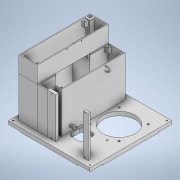
# Autodesk Inventor part: Spód
Saved by Autodesk Inventor 2022 (Build 260153000, 153)
## iProperties
Created: 2022-07-08
Part Number: Spód
Material: Ogólny
Document SubType Name: Modeling
Designer: kosak
Density: 1 g/cm^3
Appearance: Domyślna
Mass: 628.246 g
Surface Area: 3320.76 cm^2
Volume: 628.246 cm^3
Author: kosak
## iProperties of the stored document Base_Drukowanie 3D.ipt
Created: 2022-07-14
Part Number: Base_Drukowanie 3D
Material: Ogólny
Document SubType Name: Modeling
Designer: kosak
Density: 1 g/cm^3
Appearance: Domyślna
Author: kosak
Autodesk Inventor part; units mm, degrees
(part 1 of 2)
ref_plane "YZ Plane" through (0, 0, 0) normal (1, 0, 0) x (0, 1, 0)
ref_plane "XZ Plane" through (0, 0, 0) normal (0, 1, 0) x (-1, 0, 0)
ref_plane "XY Plane" through (0, 0, 0) normal (0, 0, 1) x (1, 0, 0)
sketch "Podstawa" plane through (0, 0, 0) normal (0, 1, 0) x (-1, 0, 0)
  line L0 (0, 0) -> (200, 0)
  line L1 (200, 0) -> (200, -200)
  line L2 (200, -200) -> (0, -200)
  line L3 (0, -200) -> (0, 0)
  dimension "d0" = 200
  dimension "d1" = 200
  constraints: 8 end point, 2 parallel, 1 horizontal, 1 perpendicular
  measures "d0" distance of L1.end L2.end
  measures "d1" distance of L0.end L1.end
extrude "Wyciągnięcie proste1" add sketch "Podstawa" against normal blind 10
ref_plane "Płaszczyzna konstrukcyjna3" through (0, 0, 0) normal (0, 1, 0) x (1, 0, 0)
sketch "Obrys" plane through (0, 0, 0) normal (0, 1, 0) x (1, 0, 0)
  line L0 (-200, 200) -> (0, 200) projected
  line L1 (0, 200) -> (0, 0) projected
  line L2 (-200, 200) -> (0, 200)
  line L3 (0, 200) -> (0, 0)
  line L4 (0, 0) -> (-200, 0)
  line L5 (-200, 0) -> (-200, 200)
  line L6 (-190, 190) -> (-10, 190)
  line L7 (-10, 190) -> (-10, 10)
  line L8 (-10, 10) -> (-190, 10)
  line L9 (-190, 10) -> (-190, 190)
  line L10 (-200, 0) -> (-200, 200) projected
  line L11 (-190, 190) -> (-100, 190)
  line L12 (-100, 190) -> (-96.5, 190)
  line L13 (-100, 190) -> (-103.5, 190)
  line L14 (-96.5, 190) -> (-94.2905, 190)
  line L15 (-103.5, 190) -> (-106.0324, 190)
  line L16 (-96.5, 190) -> (-103.5, 190)
  line L17 (-103.5, 190) -> (-103.5, 10)
  line L18 (-103.5, 10) -> (-96.5, 10)
  line L19 (-96.5, 10) -> (-96.5, 190)
  dimension "d5" = 10
  constraints: 34 end point, 6 parallel, 5 point on line, 3 perpendicular, 2 horizontal, 1 midpoint, 3 other
  measures "d5" distance between parallel lines of L5 L9
extrude "Wyciągnięcie proste2" [suppressed]
sketch "Podstawa - kanał powietrzny" plane through (0, 0, 0) normal (0, 1, 0) x (1, 0, 0)
  line L0 (-187, 13) -> (-187, 187)
  line L1 (-187, 187) -> (-100, 187)
  line L2 (-95.5, 13) -> (-187, 13)
  line L3 (-187, 187) -> (-142.5, 187)
  line L4 (-142.5, 187) -> (-142.5, 142.5)
  line L5 (-142.5, 142.5) -> (-187, 142.5)
  line L6 (-187, 142.5) -> (-187, 187)
  line L7 (-187, 13) -> (-142.5, 13)
  line L8 (-142.5, 13) -> (-142.5, 57.5)
  line L9 (-142.5, 57.5) -> (-187, 57.5)
  line L10 (-187, 57.5) -> (-187, 13)
  line L11 (-185, 185) -> (-144.5, 185)
  line L12 (-144.5, 185) -> (-144.5, 144.5)
  line L13 (-144.5, 144.5) -> (-185, 144.5)
  line L14 (-185, 144.5) -> (-185, 185)
  line L15 (-185, 55.5) -> (-144.5, 55.5)
  line L16 (-144.5, 55.5) -> (-144.5, 15)
  line L17 (-144.5, 15) -> (-185, 15)
  line L18 (-185, 15) -> (-185, 55.5)
  line L19 (-190, 190) -> (-190, 10) projected
  line L20 (-190, -20.8628) -> (-103.5, -20.8628)
  line L21 (-10, 10) -> (-190, 10) projected
  line L22 (-103.5, 10) -> (-103.5, 190)
  line L23 (-10, 190) -> (-190, 190) projected
  line L24 (-97.8, 10) -> (-189, 10)
  line L25 (-187, 13) -> (-10, 13)
  line L26 (-200, 0) -> (-200, 200) projected
  line L27 (-200, 200) -> (0, 200) projected
  line L28 (0, 200) -> (0, 0) projected
  line L29 (0, 0) -> (-200, 0) projected
  point P0 (-142.5, 187)
  point P1 (-142.5, 13)
  point P2 (-142.5, 13)
  dimension "d23" = 44.5
  dimension "d24" = 44.5
  dimension "d25" = 44.5
  dimension "d27" = 2
  dimension "d28" = 2
  dimension "d34" = 86.5
  dimension "d132" = 44.5
  constraints: 46 end point, 10 parallel, 5 perpendicular, 3 horizontal, 3 point on line, 1 collinear, 6 other
  measures "d23" distance of L4.end L5.end
  measures "d24" distance of L3.end L4.end
  measures "d25" distance of L9.end L8.end
  measures "d27" distance between parallel lines of L6 L14
  measures "d28" distance between parallel lines of L9 L15
  measures "d34" distance of L20.start L20.end
  measures "d132" distance between parallel lines of L9 L2
extrude "Wyciągnięcie proste5" add sketch "Podstawa - kanał powietrzny" along normal blind 100 and the other way blind 10 contours L0 L9 L8 L2 | L0 L1 L4 L5
sketch "Szkic7" plane through (0, 0, 0) normal (0, 1, 0) x (1, 0, 0)
  line L0 (-185, 144.5) -> (-144.5, 144.5) projected
  line L1 (-144.5, 144.5) -> (-144.5, 185) projected
  line L2 (-144.5, 185) -> (-185, 185) projected
  line L3 (-185, 185) -> (-185, 144.5) projected
  line L4 (-187, 142.5) -> (-187, 187) projected
  line L5 (-187, 187) -> (-142.5, 187) projected
  line L6 (-142.5, 187) -> (-142.5, 142.5) projected
  line L7 (-142.5, 142.5) -> (-187, 142.5) projected
  line L8 (-185, 15) -> (-144.5, 15) projected
  line L9 (-144.5, 15) -> (-144.5, 55.5) projected
  line L10 (-144.5, 55.5) -> (-185, 55.5) projected
  line L11 (-185, 55.5) -> (-185, 15) projected
  line L12 (-142.5, 57.5) -> (-142.5, 13) projected
  line L13 (-187, 13) -> (-187, 57.5) projected
  line L14 (-187, 57.5) -> (-142.5, 57.5) projected
  line L15 (-187, 13) -> (-187, 187)
  line L16 (-187, 187) -> (-100.8544, 187)
  line L17 (-100.8544, 13) -> (-187, 13)
  line L18 (-184.5, 142.5) -> (-184.5, 57.5)
  line L19 (-100.8544, 187) -> (-100.8544, 13)
  line L20 (-103.5, 10) -> (-96.5, 10) projected
  line L21 (-103.5, 13) -> (-100.8544, 13)
  line L22 (-103.5, 187) -> (-100.8544, 187)
  line L23 (-142.5, 142.5) -> (-187, 142.5) projected
  line L24 (-184.5, 142.5) -> (-142.5, 142.5)
  line L25 (-142.5, 142.5) -> (-142.5, 187)
  line L26 (-100.8544, 187) -> (-100.8544, 13)
  line L27 (-187, 57.5) -> (-142.5, 57.5) projected
  line L28 (-142.5, 57.5) -> (-184.5, 57.5)
  line L29 (-142.5, 13) -> (-187, 13) projected
  line L30 (-187, 13) -> (-142.5, 13) projected
  line L31 (-200, 0) -> (-200, 200) projected
  line L32 (-200, 200) -> (0, 200) projected
  line L33 (0, 200) -> (0, 0) projected
  line L34 (0, 0) -> (-200, 0) projected
  point P0 (-142.5, 13)
  point P1 (-142.5, 187)
  point P2 (-187, 57.5)
  constraints: 22 end point, 4 collinear, 4 point on line, 1 perpendicular
sketch "Otwory spód - kanał pow." plane through (0, -10, 0) normal (0, -1, 0) x (1, 0, 0)
  line L0 (-185, -144.5) -> (-144.5, -144.5) projected
  line L1 (-185, -185) -> (-185, -144.5) projected
  line L2 (-144.5, -185) -> (-185, -185) projected
  line L3 (-144.5, -144.5) -> (-144.5, -185) projected
  line L4 (-185, -55.5) -> (-185, -15) projected
  line L5 (-144.5, -55.5) -> (-185, -55.5) projected
  line L6 (-185, -15) -> (-144.5, -15) projected
  line L7 (-144.5, -15) -> (-144.5, -55.5) projected
  line L8 (-144.5, -185) -> (-185, -185) projected
  line L9 (-185, -185) -> (-144.5, -185)
  line L10 (-144.5, -185) -> (-144.5, -144.5)
  line L11 (-144.5, -144.5) -> (-185, -144.5)
  line L12 (-185, -144.5) -> (-185, -185)
  line L13 (-185, -55.5) -> (-144.5, -55.5) projected
  line L14 (-185, -55.5) -> (-144.5, -55.5)
  line L15 (-144.5, -55.5) -> (-144.5, -15)
  line L16 (-144.5, -15) -> (-185, -15)
  line L17 (-185, -15) -> (-185, -55.5)
  constraints: 16 end point, 4 parallel, 2 horizontal, 2 perpendicular
extrude "Otwory - spód" cut sketch "Otwory spód - kanał pow." against normal blind 10
ref_plane "Płaszczyzna konstrukcyjna4" through (-189, 0, -188) normal (0, 0, 1) x (1, 0, 0)
extrude "Wyciągnięcie proste18" add sketch "Szkic7" along normal blind 100 separate body contours L7 L18 L14 L15 | L7 L6 L16 L19 L17 L12 L14 L18 | L14 L12 L17 L13 | L11 L10 L9 L8
sketch "Szkic34" plane through (-142.5, 0, -187) normal (0, 0, -1) x (-1, 0, 0)
  line L0 (44.5, 0) -> (44.5, 100) projected
  line L1 (-142.5, 0.5) -> (57.5, 0.5) projected
  line L2 (44.5, 0.5) -> (32.5, 0.5)
  line L3 (32.5, 0.5) -> (32.5, 12.5)
  line L4 (32.5, 12.5) -> (44.5, 12.5)
  line L5 (44.5, 12.5) -> (44.5, 0.5)
  point P0 (-142.5, 0)
  point P1 (42.5, 201)
  point P2 (44.3955, 10.5)
  point P3 (32.5, 0.5)
  point P4 (44.5, 140)
  point P5 (44.5, 12.5)
  point P6 (44.5, 1)
  point P7 (44.5, 12.5)
  dimension "d113" = 12
  dimension "d114" = 12
  constraints: 8 end point, 2 parallel, 1 horizontal, 1 perpendicular, 1 point on line, 2 other
  measures "d113" distance of L3.end L4.end
  measures "d114" distance of L2.end L3.end
extrude "Kanał wodny - mały spód" add sketch "Szkic34" against normal blind 42.5 bodies 1
sketch "Szkic33" plane through (-142.5, 0, -187) normal (0, 0, -1) x (-1, 0, 0)
  line L0 (-142.5, 0.5) -> (57.5, 0.5) projected
  line L1 (44.5, 0) -> (44.5, 100) projected
  line L2 (47.5, 0.5) -> (-132.5, 0.5) projected
  line L3 (-132.5, 0.5) -> (47.5, 0.5) projected
  line L4 (44.5, 0.5) -> (32.5, 0.5)
  line L5 (32.5, 0.5) -> (32.5, 12.5)
  line L6 (32.5, 12.5) -> (44.5, 12.5)
  line L7 (44.5, 12.5) -> (44.5, 0.5)
  line L8 (42.5, 10.5) -> (34.5, 10.5)
  line L9 (34.5, 10.5) -> (34.5, 2.5)
  line L10 (34.5, 2.5) -> (42.5, 2.5)
  line L11 (42.5, 2.5) -> (42.5, 10.5)
  point P0 (-142.5, 0)
  point P1 (42.5, 201)
  point P2 (-43, 0.5)
  point P3 (44.5, 140)
  point P4 (44.5, 1)
  dimension "d108" = 12
  dimension "d109" = 12
  dimension "d110" = 2
  constraints: 16 end point, 4 parallel, 2 perpendicular, 1 horizontal, 1 point on line, 5 other
  measures "d108" distance of L5.end L6.end
  measures "d109" distance of L4.end L5.end
  measures "d110" distance between parallel lines of L6 L8
extrude "Kanał wodny - mały, spód" cut sketch "Szkic33" against normal blind 42.5 contours L11 L10 L9 L8 bodies 1
sketch "Szkic39" plane through (0, 100, 0) normal (0, 1, 0) x (1, 0, 0)
  line L0 (-144.5, 55.5) -> (-185, 55.5) projected
  line L1 (-185, 15) -> (-144.5, 15) projected
  line L2 (-185, 55.5) -> (-144.5, 55.5)
  line L3 (-144.5, 55.5) -> (-144.5, 15)
  line L4 (-144.5, 15) -> (-185, 15)
  line L5 (-185, 15) -> (-185, 55.5)
  point P0 (0, 0)
  point P1 (-170, 15)
  point P2 (-170, 15)
  constraints: 8 end point, 2 parallel, 1 horizontal, 1 perpendicular
extrude "Wyciągnięcie proste30" cut sketch "Szkic39" against normal blind 110 bodies 2
ref_plane "Płaszczyzna konstrukcyjna10" through (-164.75, 100, -15) normal (0, 1, 0) x (1, 0, 0)
sketch "Szkic40" plane through (-164.75, 100, -15) normal (0, 1, 0) x (1, 0, 0)
  line L0 (-22.25, 42.5) -> (-22.25, -2) projected
  line L1 (22.25, 127.5) -> (22.25, 172) projected
  line L2 (-22.25, -2) -> (22.25, -2)
  line L3 (22.25, -2) -> (22.25, 172)
  line L4 (22.25, 172) -> (-22.25, 172)
  line L5 (-22.25, 172) -> (-22.25, -2)
  point P0 (164.75, -15)
  constraints: 8 end point, 2 parallel, 1 horizontal, 1 perpendicular
extrude "Wyciągnięcie proste31" add sketch "Szkic40" along normal blind 40 bodies 2
sketch "Szkic41" plane through (-187, 0, -13) normal (0, 0, 1) x (1, 0, 0)
  line L0 (0, 140) -> (44.5, 140) projected
  line L1 (44.5, 100) -> (44.5, 140) projected
  line L2 (0, 100) -> (44.5, 100) projected
  line L3 (0, 102) -> (42.5, 102)
  line L4 (42.5, 102) -> (42.5, 138)
  line L5 (42.5, 138) -> (0, 138)
  line L6 (0, 138) -> (2, 138)
  line L7 (2, 138) -> (2, 102)
  line L8 (42.5, 102) -> (2, 102)
  line L9 (2, 102) -> (2, 138)
  line L10 (2, 138) -> (42.5, 138)
  line L11 (42.5, 138) -> (42.5, 102)
  point P0 (187, 0)
  dimension "d137" = 2
  dimension "d138" = 2
  constraints: 18 end point, 2 parallel, 2 perpendicular, 2 point on line, 1 horizontal, 2 other
  measures "d137" distance between parallel lines of L2 L3
  measures "d138" distance of L5.end L6.end
extrude "Wyciągnięcie proste32" cut sketch "Szkic41" against normal blind 172 bodies 2
sketch "Szkic42" plane through (-185, 102, -13) normal (0, 1, 0) x (1, 0, 0)
  line L0 (40.5, 2) -> (0, 2) projected
  line L1 (0, 0) -> (0, 172) projected
  line L2 (40.5, 0) -> (40.5, 172) projected
  line L3 (0, 42.5) -> (40.5, 42.5) projected
  line L4 (40.5, 42.5) -> (0, 42.5) projected
  line L5 (40.5, 2) -> (40.5, 42.5) projected
  line L6 (0, 42.5) -> (40.5, 42.5)
  line L7 (40.5, 42.5) -> (40.5, 2)
  line L8 (40.5, 2) -> (0, 2)
  line L9 (0, 2) -> (0, 42.5)
  line L10 (40.5, 131.5) -> (0, 131.5) projected
  line L11 (40.5, 172) -> (0, 172) projected
  line L12 (40.5, 131.5) -> (40.5, 172) projected
  line L13 (0, 172) -> (0, 131.5) projected
  line L14 (40.5, 172) -> (0, 172)
  line L15 (0, 172) -> (0, 131.5)
  line L16 (0, 131.5) -> (40.5, 131.5)
  line L17 (40.5, 131.5) -> (40.5, 172)
  point P0 (185, -13)
  point P1 (0, 157)
  constraints: 16 end point, 4 parallel, 2 horizontal, 2 perpendicular
extrude "Wyciągnięcie proste34" cut sketch "Szkic42" against normal blind 110 contours L0 L1 L3 L2 | L10 L1 L11 L2 bodies 2
sketch "Szkic44" plane through (0, 100, 0) normal (0, 1, 0) x (1, 0, 0)
  line L0 (-144.5, 55.5) -> (-144.5, 15) projected
  line L1 (-142.5, 13) -> (-100.8544, 13) projected
  line L2 (-100.8544, 13) -> (-100.8544, 187) projected
  line L3 (-100.8544, 187) -> (-142.5, 187) projected
  line L4 (-144.5, 185) -> (-144.5, 144.5) projected
  line L5 (-144.5, 144.5) -> (-185, 144.5) projected
  line L6 (-187, 142.5) -> (-187, 13) projected
  line L7 (-185, 55.5) -> (-144.5, 55.5) projected
  line L8 (-142.5, 185) -> (-102.8544, 185)
  line L9 (-102.8544, 185) -> (-102.8544, 15)
  line L10 (-102.8544, 15) -> (-142.5, 15)
  line L11 (-142.5, 15) -> (-142.5, 55.5)
  line L12 (-142.5, 142.5) -> (-142.5, 13) projected
  line L13 (-187, 57.5) -> (-142.5, 57.5) projected
  line L14 (-185, 57.5) -> (-142.5, 57.5)
  line L15 (-142.5, 57.5) -> (-142.5, 56.1633)
  line L16 (-185, 57.5) -> (-185, 142.5)
  line L17 (-142.5, 142.5) -> (-187, 142.5) projected
  line L18 (-185, 142.5) -> (-142.5, 142.5)
  line L19 (-142.5, 142.5) -> (-142.5, 185)
  line L20 (-142.5, 187) -> (-142.5, 142.5) projected
  point P0 (0, 0)
  dimension "d149" = 2
  constraints: 18 end point, 4 point on line, 2 collinear, 1 parallel, 1 perpendicular, 2 other
  measures "d149" distance between parallel lines of L2 L9
extrude "Wyciągnięcie proste36" cut sketch "Szkic44" against normal blind 100 contours L11 L12 L19 L8 L9 L10 | L13 L16 L17 L12 bodies 2
ref_plane "Płaszczyzna konstrukcyjna18" through (-164.75, 293.9, -15) normal (0, 1, 0) x (1, 0, 0)
sketch "Szkic49" plane through (-164.75, 293.9, -15) normal (0, 1, 0) x (1, 0, 0)
  line L0 (-22.25, 160) -> (-10.25, 160) projected
  line L1 (-10.25, 160) -> (-10.25, 172) projected
  line L2 (-10.25, 172) -> (-22.25, 172) projected
  line L3 (-22.25, 172) -> (-22.25, 160) projected
  line L4 (-20.25, 170) -> (-12.25, 170)
  line L5 (-12.25, 170) -> (-12.25, 162)
  line L6 (-12.25, 162) -> (-20.25, 162)
  line L7 (-20.25, 162) -> (-20.25, 170)
  point P0 (164.75, -15)
  dimension "d162" = 2
  constraints: 8 end point, 3 other
  measures "d162" distance between parallel lines of L2 L4
sketch "Szkic50" plane through (-185, 0, -55.5) normal (0, 0, 1) x (1, 0, 0)
  line L0 (40.5, 0) -> (0, 0) projected
  line L1 (40.5, 50) -> (0, 50)
  line L2 (40.5, 50) -> (33, 50)
  line L3 (33, 50) -> (33, 48)
  line L4 (33, 48) -> (40.5, 48)
  line L5 (40.5, 48) -> (40.5, 50)
  line L6 (0, 50) -> (7.5, 50)
  line L7 (7.5, 50) -> (7.5, 48)
  line L8 (7.5, 48) -> (0, 48)
  line L9 (0, 48) -> (0, 50)
  point P0 (185, 0)
  point P1 (33, 50)
  dimension "d165" = 50
  dimension "d166" = 7.5
  dimension "d167" = 2
  dimension "d168" = 7.5
  dimension "d169" = 2
  constraints: 18 end point, 5 parallel, 2 horizontal, 2 perpendicular
  measures "d165" distance between parallel lines of L0 L1
  measures "d166" distance of L4.end L3.end
  measures "d167" distance of L3.end L2.end
  measures "d168" distance of L7.end L8.end
  measures "d169" distance of L6.end L7.end
extrude "Wyciągnięcie proste39" add sketch "Szkic50" along normal blind 7.5 bodies 2
sketch "Szkic51" plane through (-144.5, 0, -15) normal (0, 0, -1) x (-1, 0, 0)
  line L0 (-2, 0) -> (42.5, 0) projected
  line L1 (-2, 50) -> (42.5, 50)
  line L2 (0, -10) -> (0, 100) projected
  line L3 (0, 50) -> (7.5, 50)
  line L4 (7.5, 50) -> (7.5, 48)
  line L5 (7.5, 48) -> (0, 48)
  line L6 (0, 48) -> (0, 50)
  line L7 (40.5, 100) -> (40.5, -20) projected
  line L8 (40.5, 50) -> (33, 50)
  line L9 (33, 50) -> (33, 48)
  line L10 (33, 48) -> (40.5, 48)
  line L11 (40.5, 48) -> (40.5, 50)
  point P0 (-144.5, 0)
  dimension "d172" = 50
  dimension "d173" = 7.5
  dimension "d174" = 2
  dimension "d175" = 7.5
  constraints: 18 end point, 5 parallel, 5 point on line, 2 horizontal, 2 perpendicular
  measures "d172" distance between parallel lines of L0 L1
  measures "d173" distance of L4.end L5.end
  measures "d174" distance of L3.end L4.end
  measures "d175" distance of L10.end L9.end
extrude "Wyciągnięcie proste40" add sketch "Szkic51" along normal blind 7.5 contours L2 L1 L4 L5 | L10 L9 L1 L7 bodies 2
sketch "Szkic54" plane through (-185, 48, -15) normal (0, -1, 0) x (1, 0, 0)
  line L0 (0, 0) -> (15, 0) projected
  circle A0 centre (3.75, -3.75) radius 2
  line L1 (33, -40.5) -> (33, -33) projected
  line L2 (0, -40.5) -> (40.5, -40.5) projected
  circle A1 centre (36.75, -36.75) radius 2
  line L3 (33, -7.5) -> (40.5, -7.5) projected
  line L4 (40.5, 0) -> (0, 0) projected
  circle A2 centre (36.75, -3.75) radius 2
  line L5 (0, 0) -> (0, -40.5) projected
  line L6 (7.5, -40.5) -> (7.5, -33) projected
  circle A3 centre (3.75, -36.75) radius 2
  point P0 (185, 15)
  point P1 (7.5, -7.5)
  dimension "d178" = 4
  dimension "d179" = 4
  dimension "d180" = 4
  dimension "d181" = 4
  constraints: 4 centre point
  measures "d178" diameter of A0
  measures "d179" diameter of A1
  measures "d180" diameter of A2
  measures "d181" diameter of A3
extrude "Wyciągnięcie proste41" cut sketch "Szkic54" against normal blind 2 bodies 2
ref_plane "Płaszczyzna konstrukcyjna20" through (-122.6772, -10, -159.2778) normal (0, -1, 0) x (1, 0, 0)
sketch "Szkic59" plane through (-122.6772, -10, -159.2778) normal (0, -1, 0) x (1, 0, 0)
  circle A0 centre (0, 0) radius 7
  point P0 (122.6772, 159.2778)
  dimension "d627" = 14
  constraints: 1 centre point
  measures "d627" diameter of A0
extrude "Wyciągnięcie proste44" cut sketch "Szkic59" against normal blind 10 bodies 1
sketch "Szkic60" plane through (-187, 0, -13) normal (0, 0, 1) x (1, 0, 0)
  line L0 (2, 138) -> (42.5, 138) projected
  line L1 (2, 102) -> (2, 138) projected
  line L2 (42.5, 102) -> (2, 102) projected
  line L3 (42.5, 138) -> (42.5, 102) projected
  line L4 (2, 138) -> (42.5, 138)
  line L5 (42.5, 138) -> (42.5, 102)
  line L6 (42.5, 102) -> (2, 102)
  line L7 (2, 102) -> (2, 138)
  point P0 (187, 0)
  constraints: 8 end point, 2 parallel, 1 horizontal, 1 perpendicular
extrude "Wyciągnięcie proste45" add sketch "Szkic60" against normal blind 2 bodies 2
sketch "Szkic61" plane through (-164.75, 140, -15) normal (0, 1, 0) x (1, 0, 0)
  line L0 (22.25, 172) -> (-22.25, 172) projected
  line L1 (22.25, -2) -> (22.25, 172) projected
  line L2 (-22.25, 172) -> (-22.25, -2) projected
  line L3 (-22.25, -2) -> (22.25, -2) projected
  line L4 (22.25, -2) -> (22.25, 172) projected
  line L5 (22.25, 172) -> (-22.25, 172) projected
  line L6 (-20.25, 0) -> (-20.25, 158)
  line L7 (-20.25, 158) -> (-8.25, 158)
  line L8 (-8.25, 158) -> (-8.25, 170)
  line L9 (-8.25, 170) -> (20.25, 170)
  line L10 (20.25, 170) -> (20.25, 0)
  line L11 (20.25, 0) -> (-20.25, 0)
  point P0 (164.75, -15)
  point P1 (-10.25, 172)
  dimension "d211" = 2
  constraints: 12 end point, 2 other
  measures "d211" distance between parallel lines of L2 L6
extrude "Wyciągnięcie proste46" cut sketch "Szkic61" against normal blind 2 contours L6 L7 L8 L9 L10 L11 bodies 2
sketch "Szkic67" plane through (-142.5, 100, -187) normal (1, 0, 0) x (0, 0, -1)
  line L0 (-174, 0) -> (-129.5, 0) projected
  line L1 (-172, 0) -> (-172, -100) projected
  line L2 (-129.5, -100) -> (-129.5, 0) projected
  line L3 (-44.5, 0) -> (0, 0) projected
  line L4 (-2, -100) -> (-2, 0) projected
  line L5 (-44.5, 0) -> (-44.5, -100) projected
  line L6 (-129.5, 0) -> (-129.5, -100) projected
  line L7 (-172, 0) -> (-129.5, 0)
  line L8 (-129.5, 0) -> (-129.5, -2)
  line L9 (-129.5, -2) -> (-172, -2)
  line L10 (-172, -2) -> (-172, 0)
  line L11 (-44.5, -100) -> (-44.5, 0) projected
  line L12 (-2, 0) -> (-44.5, 0)
  line L13 (-44.5, 0) -> (-44.5, -2)
  line L14 (-44.5, -2) -> (-2, -2)
  line L15 (-2, -2) -> (-2, 0)
  point P0 (-187, -100)
  point P1 (-44.5, -2)
  point P2 (-2, -2)
  point P3 (-172, -2)
  point P4 (-129.5, -2)
  dimension "d233" = 2
  dimension "d234" = 2
  constraints: 16 end point, 4 parallel, 2 horizontal, 2 perpendicular, 2 point on line
  measures "d233" distance of L7.end L8.end
  measures "d234" distance of L13.end L12.end
extrude "Wyciągnięcie proste52" add sketch "Szkic67" along normal blind 2 bodies 2
sketch "Szkic71" plane through (0, 0, 0) normal (0, 1, 0) x (1, 0, 0)
  line L0 (-100.8544, 13) -> (-100.8544, 187) projected
  line L1 (-10, 190) -> (-10, 10) projected
  line L2 (-190, 190) -> (-10, 190) projected
  line L3 (-14.854, 10) -> (-14.854, 185.146)
  line L4 (-14.854, 185.146) -> (-190, 185.146)
  line L5 (-95.8544, 13) -> (-95.8544, 187)
  circle A0 centre (-20.7504, 163.5312) radius 2.25
  line L6 (-15, 170) -> (-15, 185) projected
  line L7 (-15, 185) -> (-95.8544, 185.146)
  circle A1 centre (-92.2504, 163.5312) radius 2.25
  line L8 (-20.7504, 163.5312) -> (-92.2504, 163.5312)
  line L9 (-92.2504, 163.5312) -> (-92.2504, 92.0312)
  line L10 (-20.7504, 163.5312) -> (-20.7504, 92.0312)
  line L11 (-92.2504, 127.7812) -> (-87.467, 127.7812)
  circle A2 centre (-92.2504, 92.0312) radius 2.25
  line L12 (-20.7504, 127.7812) -> (-24.6, 127.7812)
  circle A3 centre (-20.7504, 92.0312) radius 2.25
  point P0 (0, 0)
  dimension "d271" = 4.854
  dimension "d272" = 5
  dimension "d276" = 4.5
  dimension "d415" = 4.5
  dimension "d498" = 71.5
  dimension "d499" = 71.5
  dimension "d500" = 71.5
  constraints: 18 end point, 4 centre point, 3 horizontal, 2 midpoint, 2 parallel, 2 point on line, 1 vertical, 3 other
  measures "d271" distance between parallel lines of L1 L3
  measures "d272" distance between parallel lines of L0 L5
  measures "d276" diameter of A0
  measures "d415" diameter of A1
  measures "d498" distance of L8.start L8.end
  measures "d499" distance of L8.end L9.end
  measures "d500" distance of L8.start L10.end
extrude "Wyciągnięcie proste55" cut sketch "Szkic71" against normal through all bodies 1
sketch "Szkic73" plane through (-102.8544, 100, -185) normal (-1, 0, 0) x (0, 0, 1)
  line L0 (0, 0) -> (170, 0) projected
  line L1 (0, 0) -> (0, -100) projected
  line L2 (170, -100) -> (0, -100) projected
  line L3 (170, 0) -> (170, -100) projected
  line L4 (90, -38) -> (90, -63)
  line L5 (90, -63) -> (65, -63)
  line L6 (90, -63) -> (65, -63)
  line L7 (65, -63) -> (65, -38)
  line L8 (65, -38) -> (90, -38)
  line L9 (90, -38) -> (90, -63)
  line L10 (65, -63) -> (90, -63)
  line L11 (90, -63) -> (90, -65)
  line L12 (90, -65) -> (65, -65)
  line L13 (65, -65) -> (65, -63)
  line L14 (65, -65) -> (69, -65)
  line L15 (69, -65) -> (69, -63)
  line L16 (69, -63) -> (65, -63)
  line L17 (65, -63) -> (65, -65)
  line L18 (90, -65) -> (86, -65)
  line L19 (86, -65) -> (86, -63)
  line L20 (86, -63) -> (90, -63)
  line L21 (90, -63) -> (90, -65)
  line L22 (65, -38) -> (67, -38)
  line L23 (67, -38) -> (67, -63)
  line L24 (67, -63) -> (65, -63)
  line L25 (65, -63) -> (65, -38)
  line L26 (90, -38) -> (88, -38)
  line L27 (88, -38) -> (88, -63)
  line L28 (88, -63) -> (90, -63)
  line L29 (90, -63) -> (90, -38)
  line L30 (170, 0) -> (170, -100) projected
  line L31 (170, -65) -> (90, -65)
  line L32 (172, -100) -> (-2, -100) projected
  line L33 (75.4418, -100) -> (75.4418, -75.5)
  line L34 (67, -75.5) -> (88, -75.5)
  line L35 (88, -75.5) -> (88, -77.5)
  line L36 (88, -77.5) -> (67, -77.5)
  line L37 (67, -77.5) -> (67, -75.5)
  point P0 (185, -100)
  point P1 (155, -45)
  point P2 (138.2, -85)
  point P3 (69, -63)
  dimension "d288" = 37
  dimension "d289" = 25
  dimension "d290" = 25
  dimension "d296" = 80
  dimension "d385" = 2
  dimension "d386" = 4
  dimension "d387" = 4
  dimension "d390" = 2
  dimension "d391" = 2
  dimension "d505" = 80
  dimension "d596" = 24.5
  constraints: 64 end point, 15 parallel, 7 horizontal, 7 perpendicular, 4 point on line, 2 midpoint, 1 vertical
  measures "d288" distance between parallel lines of L2 L5
  measures "d289" distance of L4.start L7.end
  measures "d290" distance of L5.end L7.end
  measures "d296" distance between parallel lines of L4 L3
  measures "d385" distance of L10.end L11.end
  measures "d386" distance of L16.end L15.end
  measures "d387" distance of L19.end L20.end
  measures "d390" distance of L23.end L24.end
  measures "d391" distance of L28.end L27.end
  measures "d505" distance of L31.start L11.end
  measures "d596" distance of L33.start L33.end
sketch "Szkic74" plane through (-100.8544, 0, -13) normal (1, 0, 0) x (0, 0, -1)
  line L0 (0, 0) -> (0, 100) projected
  line L1 (0, 0) -> (0, 100) projected
  line L2 (0, 0) -> (174, 0) projected
  circle A0 centre (40.431, 13) radius 3.9
  circle A1 centre (40.431, 13) radius 4.4
  point P0 (-13, 0)
  dimension "d323" = 7.8
  constraints: 2 centre point, 1 coincident
  measures "d323" diameter of A0
extrude "Wyciągnięcie proste58" add sketch "Szkic74" along normal blind 4 contours A0 bodies 2
sketch "Szkic75" plane through (-96.8544, 13, -53.431) normal (1, 0, 0) x (0, 0, -1)
  circle A0 centre (0, 0) radius 4.4
  point P0 (-53.431, -13)
  dimension "d304" = 8.8
  constraints: 1 centre point
  measures "d304" diameter of A0
extrude "Wyciągnięcie proste59" add sketch "Szkic75" along normal blind 0.5 bodies 2
ref_plane "Płaszczyzna konstrukcyjna12" through (-96.3544, 13, -53.431) normal (1, 0, 0) x (0, 0, -1)
sketch "Szkic77" plane through (-96.3544, 13, -53.431) normal (1, 0, 0) x (0, 0, -1)
  circle A0 centre (0, 0) radius 4.4 projected
  circle A1 centre (0, 0) radius 4.4
  point P0 (-53.431, -13)
  constraints: 1 centre point, 1 coincident, 1 concentric
extrude "Wyciągnięcie proste60" add sketch "Szkic77" along normal blind 2.5 draft -11.31 bodies 2
sketch "Szkic78" plane through (-93.8544, 13, -53.431) normal (1, 0, 0) x (0, 0, -1)
  circle A0 centre (0, 0) radius 3.9
  point P0 (-53.431, -13)
  dimension "d324" = 7.8
  constraints: 1 centre point
  measures "d324" diameter of A0
extrude "Wyciągnięcie proste61" add sketch "Szkic78" along normal blind 0.5 bodies 2
sketch "Szkic79" plane through (-93.3544, 13, -53.431) normal (1, 0, 0) x (0, 0, -1)
  circle A0 centre (0, 0) radius 4.4 projected
  circle A1 centre (0, 0) radius 4.4
  point P0 (-53.431, -13)
  constraints: 1 centre point, 1 coincident, 1 concentric
extrude "Wyciągnięcie proste62" add sketch "Szkic79" along normal blind 0.5 bodies 2
ref_plane "Płaszczyzna konstrukcyjna13" through (-92.8544, 13, -53.431) normal (1, 0, 0) x (0, 0, -1)
sketch "Szkic80" plane through (-92.8544, 13, -53.431) normal (1, 0, 0) x (0, 0, -1)
  circle A0 centre (0, 0) radius 4.4 projected
  circle A1 centre (0, 0) radius 2.2
  point P0 (-53.431, -13)
  constraints: 1 centre point, 1 coincident
extrude "Krociec - pompa" add sketch "Szkic80" along normal blind 2.5 draft -11.31 contours A0 | A1 bodies 2
sketch "Szkic81" plane through (-90.3544, 13, -53.431) normal (1, 0, 0) x (0, 0, -1)
  circle A0 centre (0, 0) radius 3.9 projected
  circle A1 centre (0, 0) radius 3.9 projected
  circle A2 centre (0, 0) radius 3.25
  point P0 (-53.431, -13)
  dimension "d320" = 6.5
  constraints: 1 centre point, 1 coincident
  measures "d320" diameter of A2
extrude "Wyciągnięcie proste64" cut sketch "Szkic81" against normal blind 15 contours A2 bodies 2
ref_plane "Płaszczyzna konstrukcyjna15" through (-164.75, 58.4, -15) normal (0, 1, 0) x (1, 0, 0)
sketch "Szkic82" plane through (-164.75, 58.4, -15) normal (0, 1, 0) x (1, 0, 0)
  line L0 (-12.25, 162) -> (-20.25, 162) projected
  line L1 (-12.25, 170) -> (-12.25, 162) projected
  line L2 (-20.25, 170) -> (-12.25, 170) projected
  line L3 (-20.25, 162) -> (-20.25, 170) projected
  line L4 (-12.25, 170) -> (-20.25, 170)
  line L5 (-20.25, 170) -> (-20.25, 162)
  line L6 (-20.25, 162) -> (-12.25, 162)
  line L7 (-12.25, 162) -> (-12.25, 170)
  constraints: 8 end point, 2 parallel, 1 horizontal, 1 perpendicular
sketch "Szkic72" plane through (0, 0, 0) normal (0, 1, 0) x (1, 0, 0)
  line L0 (-10, 190) -> (-190, 190) projected
  line L1 (-37.35, 190) -> (-37.35, 87.781)
  line L2 (-16.5, 10) -> (-16.5, 183.5)
  line L3 (-10, 10) -> (-10, 190) projected
  line L4 (-10, 79.531) -> (-37.35, 79.531)
  line L5 (-37.35, 87.781) -> (-37.35, 79.531)
  circle A0 centre (-37.35, 79.531) radius 1.5
  circle A1 centre (-37.35, 34.531) radius 1.5
  point P0 (0, 0)
  dimension "d279" = 102.219
  dimension "d281" = 27.35
  dimension "d282" = 8.25
  dimension "d283" = 3
  dimension "d285" = 3
  dimension "d294" = 45
  dimension "d295" = 27.35
  constraints: 8 end point, 2 centre point, 2 point on line, 2 vertical, 1 coincident, 1 perpendicular
  measures "d279" distance of L1.start L1.end
  measures "d281" distance of L4.end L4.start
  measures "d282" distance of L1.end L4.end
  measures "d283" diameter of A0
  measures "d285" diameter of A1
  measures "d294" distance of L4.end A1.centre
  measures "d295" distance from line of L3 A1.centre
extrude "Otwory - pompa zew" cut sketch "Szkic72" against normal blind 10 contours A0 L4 L5 | L5 L4 A0 | A1 bodies 1
sketch "Szkic87" plane through (0, 100, 0) normal (0, 1, 0) x (1, 0, 0)
  line L0 (-142.5, 13) -> (-100.8544, 13) projected
  line L1 (-100.8544, 13) -> (-100.8544, 187) projected
  line L2 (-100.8544, 13) -> (-118.8544, 13)
  line L3 (-118.8544, 13) -> (-118.8544, 33)
  line L4 (-118.8544, 33) -> (-100.8544, 33)
  line L5 (-100.8544, 33) -> (-100.8544, 13)
  point P0 (0, 0)
  point P1 (-100.8544, 33)
  point P2 (-118.8544, 13)
  dimension "d342" = 18
  dimension "d343" = 20
  constraints: 8 end point, 2 parallel, 1 horizontal, 1 perpendicular
  measures "d342" distance of L3.end L4.end
  measures "d343" distance of L2.end L3.end
extrude "Wyciągnięcie proste68" add sketch "Szkic87" against normal blind 100 bodies 2
sketch "Szkic88" plane through (0, 100, 0) normal (0, 1, 0) x (1, 0, 0)
  line L0 (-118.8544, 33) -> (-118.8544, 15) projected
  line L1 (-102.8544, 33) -> (-118.8544, 33) projected
  line L2 (-102.8544, 31) -> (-116.8544, 31)
  line L3 (-116.8544, 31) -> (-116.8544, 18)
  line L4 (-100.8544, 13) -> (-100.8544, 187) projected
  line L5 (-116.8544, 31) -> (-100.8544, 31)
  line L6 (-100.8544, 31) -> (-100.8544, 13)
  line L7 (-100.8544, 13) -> (-116.8544, 13)
  line L8 (-116.8544, 13) -> (-116.8544, 31)
  point P0 (0, 0)
  dimension "d346" = 2
  constraints: 12 end point, 2 parallel, 1 horizontal, 1 perpendicular, 1 other
  measures "d346" distance between parallel lines of L1 L2
extrude "Wyciągnięcie proste69" cut sketch "Szkic88" against normal blind 100 bodies 2
sketch "Szkic90" plane through (0, 0, 0) normal (0, 1, 0) x (1, 0, 0)
  line L0 (-10, 10) -> (-10, 190) projected
  line L1 (-190, 10) -> (-10, 10) projected
  line L2 (-116.8544, 31) -> (-116.8544, 13) projected
  line L3 (-116.8544, 13) -> (-96.8544, 13)
  line L4 (-96.8544, 13) -> (-96.8544, 20)
  line L5 (-96.8544, 20) -> (-116.8544, 20)
  line L6 (-116.8544, 20) -> (-116.8544, 13)
  point P0 (0, 0)
  dimension "d365" = 20
  dimension "d366" = 7
  constraints: 8 end point, 2 parallel, 1 horizontal, 1 perpendicular
  measures "d365" distance of L5.end L4.end
  measures "d366" distance of L4.end L3.end
extrude "Wyciągnięcie proste71" add sketch "Szkic90" along normal blind 100 bodies 1
ref_plane "Płaszczyzna konstrukcyjna17" through (-175, 140, -175) normal (1, 0, 0) x (0, 0, -1)
ref_plane "Płaszczyzna konstrukcyjna19" through (-170.4, 140, -175) normal (1, 0, 0) x (0, 0, -1)
sketch "Szkic93" plane through (-100.8544, 0, -187) normal (1, 0, 0) x (0, 0, -1)
  line L0 (-49.5921, 97.7483) -> (-47.5921, 97.7483)
  line L1 (-47.5921, 97.7483) -> (-47.5921, 95.7483)
  line L2 (-47.5921, 95.7483) -> (-49.5921, 95.7483)
  line L3 (-49.5921, 95.7483) -> (-49.5921, 97.7483)
  line L4 (-49.5921, 95.7483) -> (-49.5921, 86.9483)
  line L5 (-49.5921, 86.9483) -> (-47.5921, 86.9483)
  line L6 (-47.5921, 86.9483) -> (-47.5921, 84.9483)
  line L7 (-47.5921, 84.9483) -> (-49.5921, 84.9483)
  line L8 (-49.5921, 84.9483) -> (-49.5921, 86.9483)
  point P0 (-187, 0)
  dimension "d377" = 2
  dimension "d378" = 2
  dimension "d379" = 8.8
  dimension "d380" = 2
  constraints: 18 end point, 4 parallel, 2 horizontal, 2 perpendicular, 1 vertical
  measures "d377" distance of L1.end L2.end
  measures "d378" distance of L0.end L1.end
  measures "d379" distance of L2.end L4.end
  measures "d380" distance of L5.end L6.end
extrude "Wyciągnięcie proste73" add sketch "Szkic93" along normal blind 4.6 bodies 2
sketch "Szkic94" plane through (-96.2544, 0, -187) normal (1, 0, 0) x (0, 0, -1)
  line L0 (-47.5921, 95.7483) -> (-47.5921, 97.7483) projected
  line L1 (-49.5921, 97.7483) -> (-49.5921, 95.7483) projected
  line L2 (-47.5921, 95.7483) -> (-49.5921, 95.7483)
  line L3 (-49.5921, 95.7483) -> (-49.5921, 97.7483)
  line L4 (-49.5921, 97.7483) -> (-47.5921, 97.7483)
  line L5 (-47.5921, 97.7483) -> (-47.5921, 95.7483)
  line L6 (-48.5921, 95.7483) -> (-48.5921, 91.3483)
  line L7 (-48.5921, 91.3483) -> (-47.2595, 91.3483)
  point P0 (-187, 0)
  dimension "d383" = 4.4
  constraints: 12 end point, 2 horizontal, 2 parallel, 1 midpoint, 1 perpendicular, 1 vertical
  measures "d383" distance of L6.start L6.end
revolve "Obrót2" add sketch "Szkic94" angle 180 about axis through (-96.2544, 91.3483, -138.4079) along (0, 0, -1) bodies 2
extrude "Wyciągnięcie proste74" add sketch "Szkic73" along normal blind 2.2 contours L11 L12 L19 L5 | L5 L15 L12 L13 bodies 2
sketch "Szkic95" plane through (-102.8544, 0, -185) normal (-1, 0, 0) x (0, 0, 1)
  line L0 (65, 37) -> (69, 37) projected
  line L1 (65, 37) -> (67, 37)
  line L2 (67, 37) -> (67, 62)
  line L3 (67, 62) -> (65, 62)
  line L4 (65, 62) -> (65, 37)
  line L5 (86, 37) -> (90, 37) projected
  line L6 (90, 37) -> (88, 37)
  line L7 (88, 37) -> (88, 62)
  line L8 (88, 62) -> (90, 62)
  line L9 (90, 62) -> (90, 37)
  line L10 (152, 0) -> (0, 0) projected
  point P0 (185, 0)
  dimension "d392" = 2
  dimension "d393" = 25
  dimension "d394" = 2
  dimension "d395" = 25
  constraints: 16 end point, 4 parallel, 2 horizontal, 2 perpendicular
  measures "d392" distance of L3.end L2.end
  measures "d393" distance of L2.end L1.end
  measures "d394" distance of L7.end L8.end
  measures "d395" distance of L6.end L7.end
extrude "Wyciągnięcie proste75" add sketch "Szkic95" along normal blind 1.2 bodies 2
ref_plane "Płaszczyzna konstrukcyjna14" through (-104.0544, 0, -185) normal (-1, 0, 0) x (0, 0, 1)
sketch "Szkic96" plane through (-104.0544, 0, -185) normal (-1, 0, 0) x (0, 0, 1)
  line L0 (86, 37) -> (88, 37) projected
  line L1 (90, 62) -> (90, 35) projected
  line L2 (88, 37) -> (90, 37)
  line L3 (90, 37) -> (90, 62)
  line L4 (90, 62) -> (88, 62)
  line L5 (88, 62) -> (88, 37)
  point P0 (185, 0)
  constraints: 8 end point, 2 parallel, 1 horizontal, 1 perpendicular
extrude "Wyciągnięcie proste76" add sketch "Szkic96" along normal blind 1 bodies 2
sketch "Szkic97" plane through (-102.8544, 62, -95) normal (0, 1, 0) x (1, 0, 0)
  line L0 (0, 2) -> (0, 0) projected
  line L1 (0, 2) -> (-2.2, 2) projected
  line L2 (-2.2, 0) -> (-2.2, 2) projected
  line L3 (0, 0) -> (-2.2, 0) projected
  line L4 (0, 2) -> (-2.2, 2) projected
  line L5 (-2.2, 2) -> (-1.1, 2)
  line L6 (-2.2, 2) -> (-2.2, 4)
  line L7 (-2.2, 4) -> (-1.1, 2)
  line L8 (-2.2, 21) -> (-2.2, 25) projected
  line L9 (-2.2, 25) -> (-2.2, 21)
  line L10 (0, 23) -> (-1.2, 23) projected
  line L11 (-2.2, 21) -> (-1.2, 23)
  line L12 (-1.2, 25) -> (-2.2, 25)
  line L13 (2, -64) -> (2, 92) projected
  line L14 (-1.2, 25) -> (-1.2, 23)
  point P0 (102.8544, -95)
  point P1 (-1.1, 2)
  dimension "d401" = 2
  dimension "d413" = 4
  constraints: 14 end point, 2 vertical, 1 midpoint, 1 perpendicular, 1 point on line
  measures "d401" distance of L1.end L6.end
  measures "d413" distance of L8.end L9.end
extrude "Wyciągnięcie proste77" add sketch "Szkic97" against normal blind 25 contours L1 L6 L7 | L8 L12 L14 L11 bodies 2
fillet "Zaokrąglenie2" radius 2 2 edges at (-103.9544, 49.5, -97) (-104.0544, 49.5, -118)
fillet "Zaokrąglenie6" radius 3 2 edges at (-105.0544, 48.5, -95) (-105.0544, 48.5, -120)
sketch "Szkic99" plane through (0, 100, 0) normal (0, 1, 0) x (1, 0, 0)
  line L0 (-102.8544, 185) -> (-102.8544, 33) projected
  line L1 (-102.8544, 185) -> (-110.0544, 185)
  line L2 (-110.0544, 185) -> (-110.0544, 177.8)
  line L3 (-110.0544, 177.8) -> (-102.8544, 177.8)
  line L4 (-102.8544, 177.8) -> (-102.8544, 185)
  line L5 (-121.6772, 185) -> (-121.6772, 181.0337)
  line L6 (-140.5, 185) -> (-140.5, 177.8)
  line L7 (-140.5, 185) -> (-133.3, 185)
  line L8 (-133.3, 185) -> (-133.3, 177.8)
  line L9 (-133.3, 177.8) -> (-140.5, 177.8)
  line L10 (-187, 13) -> (-142.5, 13) projected
  line L11 (-142.5, 13) -> (-142.5, 100)
  line L12 (-142.5, 137.4079) -> (-142.5, 62.5921) projected
  line L13 (-142.5, 100) -> (-138, 100)
  line L14 (-140.5, 15) -> (-133.3, 15)
  line L15 (-133.3, 15) -> (-133.3, 22.2)
  line L16 (-133.3, 22.2) -> (-140.5, 22.2)
  line L17 (-140.5, 15) -> (-140.5, 22.2)
  line L18 (-102.8544, 177.8) -> (-102.8544, 109)
  line L19 (-102.8544, 109) -> (-110.2415, 109)
  line L20 (-102.8544, 33) -> (-110.0544, 33)
  line L21 (-110.0544, 33) -> (-110.0544, 40.2)
  line L22 (-110.0544, 40.2) -> (-102.8544, 40.2)
  point P0 (0, 0)
  point P1 (-102.8544, 177.8)
  point P2 (-102.8544, 40.2)
  dimension "d416" = 7.2
  dimension "d417" = 7.2
  dimension "d431" = 87
  constraints: 40 end point, 11 symmetric about line, 3 horizontal, 2 midpoint, 2 parallel, 1 perpendicular, 1 vertical
  measures "d416" distance of L3.end L2.end
  measures "d417" distance of L2.end L1.end
  measures "d431" distance of L10.end L11.end
extrude "Wyciągnięcie proste79" add sketch "Szkic99" against normal blind 15 bodies 2
sketch "Szkic100" plane through (0, 100, 0) normal (0, 1, 0) x (1, 0, 0)
  circle A0 centre (-107.3544, 180.5) radius 1.5
  line L0 (-110.0544, 177.8) -> (-102.8544, 177.8) projected
  line L1 (-110.0544, 185) -> (-110.0544, 177.8) projected
  line L2 (-108.8544, 185) -> (-108.8544, 179)
  line L3 (-108.8544, 179) -> (-105.0544, 179)
  line L4 (-100.8544, 187) -> (-142.5, 187) projected
  line L5 (-121.6772, 187) -> (-121.6772, 181.1)
  circle A1 centre (-136, 180.5) radius 1.5
  line L6 (-187, 13) -> (-142.5, 13) projected
  line L7 (-142.5, 13) -> (-142.5, 100)
  line L8 (-142.5, 137.4079) -> (-142.5, 62.5921) projected
  line L9 (-142.5, 100) -> (-139.5868, 100)
  circle A2 centre (-136, 19.5) radius 1.5
  line L10 (-102.8544, 177.8) -> (-102.8544, 40.2) projected
  line L11 (-102.8544, 177.8) -> (-102.8544, 109)
  line L12 (-102.8544, 109) -> (-107.1544, 109)
  circle A3 centre (-107.3544, 37.5) radius 1.5
  line L13 (-102.8544, 177.8) -> (-102.8544, 182.3)
  point P0 (0, 0)
  dimension "d420" = 3
  dimension "d430" = 1.2
  dimension "d432" = 87
  constraints: 16 end point, 4 centre point, 3 midpoint, 3 symmetric about line, 2 horizontal, 2 tangent, 1 vertical, 4 other
  measures "d420" diameter of A0
  measures "d430" distance between parallel lines of L1 L2
  measures "d432" distance of L6.end L7.end
extrude "Wyciągnięcie proste80" cut sketch "Szkic100" against normal blind 10 contours A0 | A1 | A2 | A3 bodies 2
sketch "Szkic101" plane through (0, 100, 0) normal (0, 1, 0) x (1, 0, 0)
  line L0 (-140.5, 22.2) -> (-133.3, 22.2) projected
  line L1 (-133.3, 22.2) -> (-133.3, 15) projected
  line L2 (-140.5, 22.2) -> (-133.3, 22.2)
  line L3 (-133.3, 22.2) -> (-133.3, 15)
  line L4 (-133.3, 15) -> (-140.5, 15)
  line L5 (-140.5, 15) -> (-140.5, 22.2)
  line L6 (-133.3, 177.8) -> (-140.5, 177.8) projected
  line L7 (-140.5, 185) -> (-142.5, 185) projected
  line L8 (-133.3, 177.8) -> (-140.5, 177.8)
  line L9 (-140.5, 177.8) -> (-140.5, 185)
  line L10 (-140.5, 185) -> (-133.3, 185)
  line L11 (-133.3, 185) -> (-133.3, 177.8)
  line L12 (-110.0544, 177.8) -> (-110.0544, 185) projected
  line L13 (-110.0544, 177.8) -> (-102.8544, 177.8)
  line L14 (-102.8544, 177.8) -> (-102.8544, 185)
  line L15 (-102.8544, 185) -> (-110.0544, 185)
  line L16 (-110.0544, 185) -> (-110.0544, 177.8)
  line L17 (-100.8544, 187) -> (-142.5, 187) projected
  line L18 (-100.8544, 187) -> (-100.8544, 109)
  line L19 (-100.8544, 31) -> (-100.8544, 187) projected
  line L20 (-100.8544, 109) -> (-110.4695, 109)
  line L21 (-110.0544, 40.2) -> (-110.0544, 33)
  line L22 (-110.0544, 40.2) -> (-102.8544, 40.2)
  line L23 (-102.8544, 40.2) -> (-102.8544, 33)
  line L24 (-102.8544, 33) -> (-110.0544, 33)
  point P0 (0, 0)
  constraints: 36 end point, 6 parallel, 5 symmetric about line, 4 horizontal, 3 perpendicular, 1 midpoint
extrude "Wyciągnięcie proste81" cut sketch "Szkic101" against normal blind 3 bodies 2
sketch "Szkic102" plane through (-164.75, 140, -15) normal (0, 1, 0) x (1, 0, 0)
  line L0 (20.25, 170) -> (13.05, 170)
  line L1 (13.05, 170) -> (13.05, 162.8)
  line L2 (13.05, 162.8) -> (20.25, 162.8)
  line L3 (20.25, 162.8) -> (20.25, 170)
  line L4 (20.25, 0) -> (-20.25, 0) projected
  line L5 (20.25, 0) -> (13.05, 0)
  line L6 (13.05, 0) -> (13.05, 7.2)
  line L7 (13.05, 7.2) -> (20.25, 7.2)
  line L8 (20.25, 7.2) -> (20.25, 0)
  line L9 (-20.25, 0) -> (-13.05, 0)
  line L10 (-13.05, 0) -> (-13.05, 7.2)
  line L11 (-13.05, 7.2) -> (-20.25, 7.2)
  line L12 (-20.25, 7.2) -> (-20.25, 0)
  line L13 (-8.25, 158) -> (-20.25, 158) projected
  line L14 (-20.25, 158) -> (-13.05, 158)
  line L15 (-13.05, 158) -> (-13.05, 150.3)
  line L16 (-13.05, 150.3) -> (-20.25, 150.3)
  line L17 (-20.25, 150.3) -> (-20.25, 158)
  point P0 (164.75, -15)
  point P1 (13.05, 0)
  point P2 (-13.05, 0)
  dimension "d441" = 7.2
  dimension "d442" = 7.2
  dimension "d443" = 7.2
  dimension "d444" = 7.2
  dimension "d445" = 7.2
  dimension "d446" = 7.2
  dimension "d447" = 7.2
  dimension "d448" = 7.7
  constraints: 32 end point, 8 parallel, 4 horizontal, 4 perpendicular
  measures "d441" distance of L2.end L1.end
  measures "d442" distance of L1.end L0.end
  measures "d443" distance of L6.end L7.end
  measures "d444" distance of L5.end L6.end
  measures "d445" distance of L11.end L10.end
  measures "d446" distance of L10.end L9.end
  measures "d447" distance of L15.end L16.end
  measures "d448" distance of L14.end L15.end
extrude "Wyciągnięcie proste82" add sketch "Szkic102" against normal blind 15 bodies 2
sketch "Szkic103" plane through (-164.75, 140, -15) normal (0, 1, 0) x (1, 0, 0)
  line L0 (-13.05, 7.2) -> (-20.25, 7.2) projected
  line L1 (-13.05, 0) -> (-13.05, 7.2) projected
  line L2 (-18.05, 6) -> (-14.25, 6)
  line L3 (-14.25, 6) -> (-14.25, 0)
  circle A0 centre (-15.75, 4.5) radius 1.5
  line L4 (-20.25, 0) -> (-13.05, 0) projected
  line L5 (-20.25, 0) -> (-5.25, 0) projected
  line L6 (-20.25, 0) -> (0, 0)
  line L7 (0, 0) -> (0, 0.9959)
  circle A1 centre (15.75, 4.5) radius 1.5
  line L8 (-20.25, 7.2) -> (-20.25, 150.3) projected
  line L9 (-20.25, 7.2) -> (-20.25, 150.3)
  line L10 (20.25, 162.8) -> (20.25, 7.2) projected
  line L11 (-20.25, 78.75) -> (-16.65, 78.75)
  circle A2 centre (-15.75, 153) radius 1.5
  line L12 (20.25, 7.2) -> (20.25, 162.8)
  line L13 (22.25, 127.5) -> (22.25, 172) projected
  line L14 (20.25, 7.2) -> (13.05, 7.2) projected
  line L15 (20.25, 7.2) -> (20.25, 85)
  line L16 (20.25, 129.5) -> (20.25, 170) projected
  line L17 (20.25, 85) -> (15.75, 85)
  circle A3 centre (15.75, 165.5) radius 1.5
  point P0 (164.75, -15)
  point P1 (20.25, 109)
  point P2 (20.25, 69)
  dimension "d451" = 1.2
  dimension "d452" = 3
  dimension "d453" = 20.25
  dimension "d473" = 77.8
  constraints: 18 end point, 4 centre point, 3 symmetric about line, 2 horizontal, 2 parallel, 2 tangent, 1 midpoint, 1 point on line, 1 vertical, 4 other
  measures "d451" distance between parallel lines of L0 L2
  measures "d452" diameter of A0
  measures "d453" distance of L4.start L6.end
  measures "d473" distance of L10.end L15.end
extrude "Wyciągnięcie proste83" cut sketch "Szkic103" against normal blind 10 contours A0 | A1 | A2 | A3 bodies 2
sketch "Szkic104" plane through (-164.75, 140, -15) normal (0, 1, 0) x (1, 0, 0)
  line L0 (-13.05, 7.2) -> (-20.25, 7.2) projected
  line L1 (-20.25, 15) -> (-20.25, 0) projected
  line L2 (-13.05, 7.2) -> (-20.25, 7.2)
  line L3 (-20.25, 7.2) -> (-20.25, 0)
  line L4 (-20.25, 0) -> (-13.05, 0)
  line L5 (-13.05, 0) -> (-13.05, 7.2)
  line L6 (13.05, 7.2) -> (13.05, 0) projected
  line L7 (-20.25, 0) -> (20.25, 0) projected
  line L8 (13.05, 7.2) -> (20.25, 7.2)
  line L9 (20.25, 7.2) -> (20.25, 0)
  line L10 (20.25, 0) -> (13.05, 0)
  line L11 (13.05, 0) -> (13.05, 7.2)
  line L12 (13.05, 170) -> (13.05, 162.8) projected
  line L13 (-20.25, 170) -> (20.25, 170) projected
  line L14 (13.05, 162.8) -> (20.25, 162.8)
  line L15 (20.25, 162.8) -> (20.25, 170)
  line L16 (20.25, 170) -> (13.05, 170)
  line L17 (13.05, 170) -> (13.05, 162.8)
  line L18 (-13.05, 150.3) -> (-13.05, 158) projected
  line L19 (-20.25, 158) -> (-13.05, 158) projected
  line L20 (-13.05, 150.3) -> (-20.25, 150.3)
  line L21 (-20.25, 150.3) -> (-20.25, 158)
  line L22 (-20.25, 158) -> (-13.05, 158)
  line L23 (-13.05, 158) -> (-13.05, 150.3)
  point P0 (164.75, -15)
  point P1 (-5.25, 0)
  constraints: 32 end point, 8 parallel, 4 horizontal, 4 perpendicular
extrude "Wyciągnięcie proste84" cut sketch "Szkic104" against normal blind 3 bodies 2
sketch "Szkic105" plane through (-133.3, 85, -22.2) normal (0, 0, -1) x (-1, 0, 0)
  line L0 (7.2, 0) -> (0, 0) projected
  line L1 (9.2, 13) -> (7.2, 13) projected
  line L2 (7.2, 0) -> (9.2, 0)
  line L3 (9.2, 0) -> (9.2, 13)
  line L4 (9.2, 13) -> (7.2, 13)
  line L5 (7.2, 13) -> (7.2, 0)
  point P0 (-133.3, -85)
  constraints: 8 end point, 2 parallel, 1 horizontal, 1 perpendicular
extrude "Wyciągnięcie proste85" add sketch "Szkic105" against normal through all bodies 2
sketch "Szkic106" plane through (-140.5, 85, -177.8) normal (0, 0, 1) x (1, 0, 0)
  line L0 (0, 15) -> (0, 13) projected
  line L1 (-2, -85) -> (-2, 15) projected
  line L2 (0, 13) -> (-2, 13)
  line L3 (-2, 13) -> (-2, -0.0383)
  line L4 (-2, -0.0383) -> (0, -0.0383)
  line L5 (0, -0.0383) -> (0, 13)
  point P0 (140.5, -85)
  constraints: 8 end point, 2 parallel, 1 horizontal, 1 perpendicular, 1 point on line
extrude "Wyciągnięcie proste86" add sketch "Szkic106" against normal through all bodies 2
extrude "Wyciągnięcie proste89" cut sketch "Szkic49" against normal blind 293 contours L4 L5 L6 L7 bodies 2
ref_plane "Płaszczyzna konstrukcyjna16" through (-185, 12.5, -185) normal (0, 1, 0) x (1, 0, 0)
sketch "Szkic110" plane through (-102.8544, 100, -185) normal (-1, 0, 0) x (0, 0, 1)
  line L0 (99.8, -17) -> (93.8, -17)
  line L1 (93.8, -11.8) -> (99.8, -11.8)
  line L2 (152, -100) -> (0, -100) projected
  line L3 (105.3831, -100) -> (105.3831, -69)
  line L4 (105.3831, -69) -> (111.3831, -69)
  line L5 (111.3831, -69) -> (111.3831, -67)
  line L6 (111.3831, -67) -> (105.3831, -67)
  line L7 (105.3831, -67) -> (105.3831, -69)
  line L8 (93.8, -11.8) -> (93.8, -13.8)
  line L9 (93.8, -13.8) -> (99.8, -13.8)
  line L10 (99.8, -15) -> (93.8, -15)
  line L11 (99.8, -11.8) -> (99.8, -13.8)
  line L12 (99.8, -15) -> (99.8, -17)
  line L13 (93.8, -17) -> (93.8, -15)
  line L14 (93.8, -13.8) -> (93.8, -11.8)
  line L15 (111.3831, -65.8) -> (105.3831, -65.8)
  line L16 (105.3831, -65.8) -> (105.3831, -63.8)
  line L17 (105.3831, -63.8) -> (111.3831, -63.8)
  line L18 (111.3831, -63.8) -> (111.3831, -65.8)
  line L19 (108.3831, -67) -> (108.3831, -65.8)
  line L20 (97.3513, -15) -> (97.3513, -13.8)
  line L21 (144.8, -15) -> (144.8, -3) projected
  line L22 (144.8, -15) -> (99.8, -15)
  point P0 (185, -100)
  dimension "d525" = 6
  dimension "d534" = 31
  dimension "d536" = 2
  dimension "d548" = 2
  dimension "d554" = 1.2
  dimension "d555" = 1.2
  dimension "d556" = 45
  dimension "d557" = 2
  dimension "d558" = 2
  constraints: 42 end point, 10 parallel, 4 horizontal, 4 perpendicular, 4 point on line, 2 midpoint, 2 vertical
  measures "d525" distance of L1.start L1.end
  measures "d534" distance of L3.start L3.end
  measures "d536" distance of L5.end L4.end
  measures "d548" distance of L15.end L16.end
  measures "d554" distance of L19.start L19.end
  measures "d555" distance of L20.start L20.end
  measures "d556" distance of L21.start L10.start
  measures "d557" distance of L8.end L1.start
  measures "d558" distance of L0.end L10.end
extrude "Wyciągnięcie proste91" add sketch "Szkic110" along normal blind 8 bodies 2
sketch "Szkic111" plane through (-102.8544, 88.2, -85.2) normal (0, 1, 0) x (1, 0, 0)
  line L0 (0, 6) -> (0, 0) projected
  circle A0 centre (-4.5, 3) radius 1.5
  line L1 (-3, 3) -> (0, 3)
  line L2 (0, 0) -> (0, 6) projected
  point P0 (102.8544, -85.2)
  point P1 (-8, 0)
  dimension "d570" = 3
  dimension "d569" = 3
  constraints: 2 end point, 1 horizontal alignment, 1 midpoint, 2 other
  measures "d569" distance of L1.start L1.end
extrude "Wyciągnięcie proste92" cut sketch "Szkic111" against normal blind 6 bodies 2
thread "Gwint25" size "M3x0.5" class "6H" standard "ANSI Metric M Profile" full length
sketch "Szkic113" plane through (-102.8544, 36.2, -73.6169) normal (0, 1, 0) x (1, 0, 0)
  line L0 (0, 0) -> (-8, 0) projected
  line L1 (0, 6) -> (0, 0) projected
  circle A0 centre (-4.5, 3) radius 1.5
  line L2 (-3, 3) -> (0, 3)
  point P0 (102.8544, -73.6169)
  dimension "d549" = 3
  dimension "d571" = 3
  constraints: 2 end point, 1 horizontal alignment, 1 midpoint, 2 other
  measures "d571" distance of L2.start L2.end
extrude "Wyciągnięcie proste94" cut sketch "Szkic113" against normal blind 7 bodies 2
thread "Gwint26" size "M3x0.5" class "6H" standard "ANSI Metric M Profile" full length